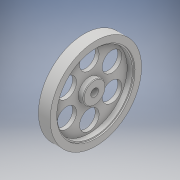
# Autodesk Inventor part: Roue
Saved by Autodesk Inventor 2018 (Build 220112000, 112)
## iProperties
Created: 2019-11-07
Part Number: Roue
Material: Generic
Document SubType Name: Modeling
Designer: hugo
Density: 1 g/cm^3
Appearance: Default
Author: hugo
Autodesk Inventor part; units mm, degrees
ref_plane "YZ Plane" through (0, 0, 0) normal (1, 0, 0) x (0, 1, 0)
ref_plane "XZ Plane" through (0, 0, 0) normal (0, 1, 0) x (-1, 0, 0)
ref_plane "XY Plane" through (0, 0, 0) normal (0, 0, 1) x (1, 0, 0)
sketch "Sketch1" plane through (0, 0, 0) normal (1, 0, 0) x (0, 1, 0)
  circle A0 centre (0, 0) radius 35
  dimension "d0" = 70
  constraints: 1 centre point, 1 coincident
  measures "d0" diameter of A0
extrude "Extrusion1" add sketch "Sketch1" along normal blind 9
sketch "Sketch2" plane through (9, 0, 0) normal (1, 0, 0) x (0, 0, -1)
  circle A0 centre (0, 0) radius 29
  circle A1 centre (0, 0) radius 35 projected
  dimension "d3" = 6
  constraints: 1 centre point, 1 coincident
  measures "d3" radial gap between concentric circles of A1 A0
extrude "Extrusion2" cut sketch "Sketch2" against normal blind 5 contours A0
sketch "Sketch3" plane through (0, 0, 0) normal (-1, 0, 0) x (0, 0, 1)
  circle A0 centre (0, 0) radius 29 projected
  circle A1 centre (0, 0) radius 30
  dimension "d14" = 1
  constraints: 1 centre point, 1 coincident
  measures "d14" radial gap between concentric circles of A1 A0
extrude "Extrusion3" cut sketch "Sketch3" against normal blind 1 contours A0 | A1
sketch "Sketch4" plane through (4, 0, 0) normal (1, 0, 0) x (0, 0, -1)
  circle A0 centre (0, 0) radius 8.5
  dimension "d8" = 17
  constraints: 1 centre point, 1 coincident
  measures "d8" diameter of A0
extrude "Extrusion4" add sketch "Sketch4" along normal blind 4
sketch "Sketch5" plane through (8, 0, 0) normal (1, 0, 0) x (0, 0, -1)
  circle A0 centre (0, 0) radius 3
  dimension "d11" = 6
  constraints: 1 centre point, 1 coincident
  measures "d11" diameter of A0
extrude "Extrusion5" cut sketch "Sketch5" against normal up to next
sketch "Sketch6" plane through (9, 0, 0) normal (1, 0, 0) x (0, 0, -1)
  circle A0 centre (0, 0) radius 29 projected
  circle A1 centre (0, 0) radius 30
  dimension "d15" = 1
  constraints: 1 centre point, 1 coincident
  measures "d15" radial gap between concentric circles of A1 A0
extrude "Extrusion6" cut sketch "Sketch6" against normal blind 1
sketch "Sketch7" plane through (4, 0, 0) normal (1, 0, 0) x (0, 0, -1)
  point P0 (0, 0)
  point P1 (20, 0)
  point P2 (10, 17.3205)
  point P3 (-10, 17.3205)
  point P4 (-20, 0)
  point P5 (-10, -17.3205)
  point P6 (10, -17.3205)
  dimension "d18" = 20
  dimension "d21" = 360
  constraints: 7 other
  measures "d18" distance of point (0, 0) point (20, 0)
hole "Hole1" at (4, 0, -20) at (4, 17.3205, -10) at (4, 17.3205, 10) at (4, 0, 20) at (4, -17.3205, 10) at (4, -17.3205, -10) direction (-1, 0, 0) diameter 15 end through all
fillet "Fillet1" radius 0.5 1 edges at (8, 0, 8.5)
equation "\"d0\" = Ar"
equation "\"d1\" = Er"
equation "\"d3\" = Dr"
equation "\"d8\" = Cr"
equation "\"d11\" = Br"
equation "\"Ar\" = 70"
equation "\"Br\" = 6"
equation "\"Cr\" = 17"
equation "\"Dr\" = 6"
equation "\"Er\" = 9"
body "Solid1"
